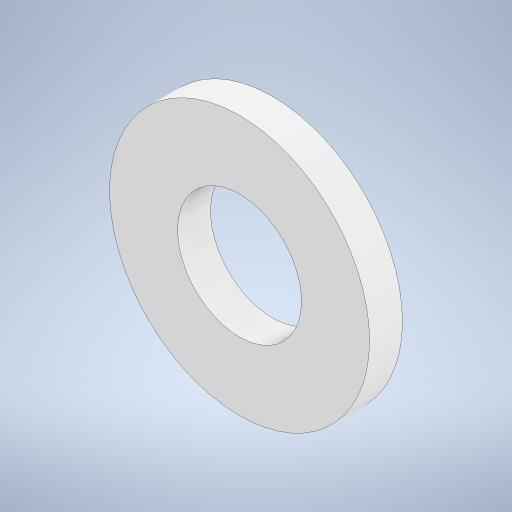
# Autodesk Inventor part: Keystone 3348
Saved by Autodesk Inventor 2024.2 (Build 282272000, 272)
## iProperties
Created: 2022-01-25
Part Number: Keystone 3348
Material: Generic
Document SubType Name: Modeling
Designer: magoo
Density: 1 g/cm^3
Appearance: Default
Description: #4 Nylon flat washer
Author: magoo
Autodesk Inventor part; units mm, degrees
ref_plane "YZ Plane" through (0, 0, 0) normal (1, 0, 0) x (0, 1, 0)
ref_plane "XZ Plane" through (0, 0, 0) normal (0, 1, 0) x (-1, 0, 0)
ref_plane "XY Plane" through (0, 0, 0) normal (0, 0, 1) x (1, 0, 0)
sketch "Sketch1" plane through (0, 0, 0) normal (0, 0, 1) x (1, 0, 0)
  circle A0 centre (0, 0) radius 1.525
  circle A1 centre (0, 0) radius 3.2
  dimension "d0" = 3.05
  dimension "d1" = 6.4
  constraints: 2 centre point, 2 coincident
  measures "d0" diameter of A0
  measures "d1" diameter of A1
extrude "Extrusion1" add sketch "Sketch1" along normal blind 0.81
body "Solid1"
